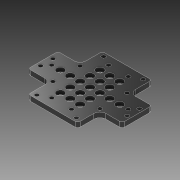
# Autodesk Inventor part: Drill Guide
Saved by Autodesk Inventor 2022 (Build 260153000, 153)
## iProperties
Created: 2021-07-10
Part Number: Drill Guide
Material: Aluminum 6061
Document SubType Name: Modeling
Designer: Max Boord
Density: 2.7 g/cm^3
Appearance: Glossy - Black
Author: Max Boord
Autodesk Inventor part; units mm, degrees
ref_plane "YZ Plane" through (0, 0, 0) normal (1, 0, 0) x (0, 1, 0)
ref_plane "XZ Plane" through (0, 0, 0) normal (0, 1, 0) x (-1, 0, 0)
ref_plane "XY Plane" through (0, 0, 0) normal (0, 0, 1) x (1, 0, 0)
sketch "Sketch1" plane through (0, 0, 0) normal (0, 1, 0) x (-1, 0, 0)
  line L0 (-25.4, -38.1) -> (25.4, -38.1) construction
  line L1 (25.4, -38.1) -> (25.4, -29.8901)
  line L2 (25.4, 38.1) -> (-25.4, 38.1) construction
  line L3 (-25.4, -29.8901) -> (-25.4, -38.1)
  line L4 (-25.4, -38.1) -> (25.4, 38.1) construction
  line L5 (25.4, -38.1) -> (-25.4, 38.1) construction
  circle A0 centre (12.7, -28.575) radius 4.7625
  circle A1 centre (0, -28.575) radius 4.7625
  circle A2 centre (-12.7, -28.575) radius 4.7625
  circle A3 centre (12.7, -15.875) radius 4.7625
  circle A4 centre (0, -15.875) radius 4.7625
  circle A5 centre (-12.7, -15.875) radius 4.7625
  circle A6 centre (12.7, -3.175) radius 4.7625
  circle A7 centre (0, -3.175) radius 4.7625
  circle A8 centre (-12.7, -3.175) radius 4.7625
  circle A9 centre (12.7, 9.525) radius 4.7625
  circle A10 centre (0, 9.525) radius 4.7625
  circle A11 centre (-12.7, 9.525) radius 4.7625
  circle A12 centre (12.7, 22.225) radius 4.7625
  circle A13 centre (0, 22.225) radius 4.7625
  circle A14 centre (-12.7, 22.225) radius 4.7625
  line L6 (47.625, -15.875) -> (47.625, 9.525) construction
  circle A15 centre (25.4, -3.175) radius 4.7625
  circle A16 centre (38.1, -3.175) radius 4.7625
  line L7 (0, -38.1) -> (0, 38.1) construction
  circle A17 centre (-25.4, -3.175) radius 4.7625
  circle A18 centre (-38.1, -3.175) radius 4.7625
  arc A19 (39.4151, -15.875) -> (25.4, -29.8901) centre (39.4151, -29.8901) ccw construction
  line L8 (25.4, 38.1) -> (25.4, 23.5401) construction
  arc A20 (25.4, 23.5401) -> (39.4151, 9.525) centre (39.4151, 23.5401) ccw construction
  line L9 (-60.325, -15.875) -> (-39.4151, -15.875) construction
  line L10 (-60.325, 9.525) -> (-39.4151, 9.525) construction
  arc A21 (-25.4, -29.8901) -> (-39.4151, -15.875) centre (-39.4151, -29.8901) ccw construction
  line L11 (-25.4, 23.5401) -> (-25.4, 38.1) construction
  arc A22 (-39.4151, 9.525) -> (-25.4, 23.5401) centre (-39.4151, 23.5401) ccw construction
  line L12 (53.975, -15.875) -> (28.575, -15.875) construction
  line L13 (25.4, -19.05) -> (25.4, -44.45) construction
  line L14 (-25.4, -44.45) -> (-25.4, -19.05) construction
  line L15 (-28.575, -15.875) -> (-39.4151, -15.875) construction
  line L16 (-25.4, 23.5401) -> (-25.4, 12.7) construction
  line L17 (-39.4151, 9.525) -> (-28.575, 9.525) construction
  line L18 (25.4, 23.5401) -> (25.4, 12.7) construction
  line L19 (28.575, 9.525) -> (53.975, 9.525) construction
  arc A23 (25.4, 12.7) -> (28.575, 9.525) centre (28.575, 12.7) ccw construction
  arc A24 (28.575, -15.875) -> (25.4, -19.05) centre (28.575, -19.05) ccw construction
  arc A25 (-25.4, -19.05) -> (-28.575, -15.875) centre (-28.575, -19.05) ccw construction
  arc A26 (-28.575, 9.525) -> (-25.4, 12.7) centre (-28.575, 12.7) ccw construction
  line L20 (39.4151, -22.225) -> (53.975, -22.225)
  line L21 (53.975, -22.225) -> (53.975, 15.875) construction
  line L22 (53.975, 15.875) -> (39.4151, 15.875)
  arc A27 (39.4151, -22.225) -> (31.75, -29.8901) centre (39.4151, -29.8901) ccw
  line L23 (31.75, -29.8901) -> (31.75, -44.45)
  line L24 (31.75, -44.45) -> (-31.75, -44.45) construction
  line L25 (-31.75, -44.45) -> (-31.75, -29.8901)
  arc A28 (-31.75, -29.8901) -> (-39.4151, -22.225) centre (-39.4151, -29.8901) ccw
  line L26 (-39.4151, -22.225) -> (-60.325, -22.225)
  line L27 (-60.325, -22.225) -> (-60.325, 15.875)
  line L28 (-60.325, 15.875) -> (-39.4151, 15.875)
  arc A29 (-39.4151, 15.875) -> (-31.75, 23.5401) centre (-39.4151, 23.5401) ccw
  line L29 (-31.75, 23.5401) -> (-31.75, 44.45)
  line L30 (-31.75, 44.45) -> (31.75, 44.45)
  line L31 (31.75, 44.45) -> (31.75, 23.5401)
  arc A30 (31.75, 23.5401) -> (39.4151, 15.875) centre (39.4151, 23.5401) ccw
  line L32 (25.4, 38.1) -> (25.4, 44.45) construction
  line L33 (-25.4, 38.1) -> (-25.4, 44.45)
  circle A31 centre (-55.5625, -3.175) radius 4.7625 construction
  circle A32 centre (49.2125, -3.175) radius 4.7625 construction
  circle A33 centre (0, -39.6875) radius 4.7625 construction
  circle A34 centre (0, 39.6875) radius 4.7625 construction
  line L34 (44.45, -17.4132) -> (44.45, -3.2681) construction
  line L35 (-50.8, -20.963) -> (-50.8, -1.2168) construction
  line L36 (-5.6388, -34.925) -> (9.5526, -34.925) construction
  line L37 (-7.9375, 34.925) -> (9.5526, 34.925) construction
  circle A35 centre (-55.5625, -3.175) radius 2.4892 construction
  circle A36 centre (0, -39.6875) radius 2.4892 construction
  circle A37 centre (49.2125, -3.175) radius 2.4892
  circle A38 centre (0, 39.6875) radius 2.4892 construction
  line L38 (33.9951, -24.4701) -> (26.3299, -16.8049) construction
  circle A39 centre (30.1625, -20.6375) radius 2.5527
  circle A40 centre (-30.1625, -20.6375) radius 2.5527
  line L39 (53.975, -3.175) -> (-60.325, -3.175) construction
  circle A41 centre (30.1625, 14.2875) radius 2.5527
  circle A42 centre (-30.1625, 14.2875) radius 2.5527
  circle A43 centre (25.4, 39.6875) radius 2.4892
  circle A44 centre (12.7, 39.6875) radius 2.4892 construction
  circle A45 centre (0, 39.6875) radius 2.4892 construction
  circle A46 centre (-12.7, 39.6875) radius 2.4892 construction
  circle A47 centre (-25.4, 39.6875) radius 2.4892
  circle A48 centre (12.7, -39.6875) radius 2.4892
  circle A49 centre (25.4, -39.6875) radius 2.4892 construction
  circle A50 centre (-12.7, -39.6875) radius 2.4892
  circle A51 centre (-25.4, -39.6875) radius 2.4892 construction
  circle A52 centre (49.2125, -11.1125) radius 2.4892 construction
  circle A53 centre (30.1625, -20.6375) radius 4.7625 construction
  circle A54 centre (49.2125, 4.7625) radius 2.4892 construction
  circle A55 centre (49.2125, 4.7625) radius 4.7625 construction
  circle A56 centre (49.2125, -11.1125) radius 4.7625 construction
  circle A57 centre (-55.5625, -11.1125) radius 2.4892
  circle A58 centre (-55.5625, -11.1125) radius 4.7625 construction
  circle A59 centre (-55.5625, 4.7625) radius 2.4892
  circle A60 centre (-55.5625, 4.7625) radius 4.7625 construction
  circle A61 centre (-12.7, 33.3375) radius 2.4892
  circle A62 centre (12.7, 33.3375) radius 2.4892
  circle A63 centre (-25.4, -46.0375) radius 2.4892
  circle A64 centre (25.4, -46.0375) radius 2.4892
  line L40 (31.75, -44.45) -> (31.75, -50.8)
  line L41 (31.75, -50.8) -> (-31.75, -50.8)
  line L42 (-31.75, -50.8) -> (-31.75, -44.45)
  line L43 (25.4, -44.45) -> (25.4, -50.8) construction
  line L44 (-25.4, -44.45) -> (-25.4, -50.8) construction
  circle A65 centre (-49.2125, -3.175) radius 2.4892
  circle A66 centre (55.5625, 4.7625) radius 2.4892
  circle A67 centre (55.5625, -11.1125) radius 2.4892
  line L45 (53.975, -22.225) -> (60.325, -22.225)
  line L46 (60.325, -22.225) -> (60.325, 15.875)
  line L47 (53.975, 15.875) -> (60.325, 15.875)
  line L48 (53.975, 9.525) -> (60.325, 9.525) construction
  line L49 (53.975, -15.875) -> (60.325, -15.875) construction
  circle A68 centre (25.4, -46.0375) radius 4.7625
  line L50 (25.4, -41.275) -> (19.287, -41.275)
  circle A69 centre (12.7, 33.3375) radius 4.7625
  line L51 (15.952, 28.575) -> (5.0903, 28.575) construction
  circle A70 centre (55.5625, 4.7625) radius 4.7625 construction
  line L52 (50.8, 8.631) -> (50.8, -0.466) construction
  point P0 (0, 0)
  point P1 (47.625, -3.175)
  point P2 (-25.4, 9.525)
  point P3 (47.625, -15.875)
  point P4 (47.625, 9.525)
  dimension "d15" = 25.4
  dimension "d0" = 50.8
  dimension "d3" = 9.525
  dimension "d6" = 12.7
  dimension "d9" = 12.7
  dimension "d18" = 12.7
  dimension "d29" = 3.175
  dimension "d30" = 6.35
  dimension "d31" = 7.6651
  dimension "d65" = 9.525
  dimension "d67" = 6.35
  dimension "d68" = 12.7
  dimension "d69" = 4.7625
  dimension "d70" = 25.4
  dimension "d71" = 6.35
  dimension "d74" = 12.7
  dimension "d89" = 4.9784
  dimension "d90" = 5.1054
  dimension "d100" = 4.9784
  dimension "d101" = 6.35
  dimension "d104" = 12.7
  dimension "d112" = 360
  dimension "d114" = 4.9784
  dimension "d126" = 9.525
  dimension "d127" = 9.525
  dimension "d128" = 9.525
  dimension "d129" = 4.9784
  dimension "d132" = 360
  dimension "d134" = 47.625
  dimension "d135" = 47.625
  dimension "d138" = 360
  dimension "d140" = 60.325
  dimension "d141" = 60.325
  dimension "d142" = 6.35
  dimension "d143" = 12.7
  constraints: 106 end point, 70 centre point, 39 tangent, 27 point on circle, 26 point on line, 20 equal radius, 18 horizontal, 13 coincident, 13 perpendicular, 13 vertical, 8 midpoint, 5 parallel, 5 symmetric about line, 4 horizontal alignment, 2 vertical alignment, 109 other
  measures "d0" distance of L2.end L2.start
  measures "d3" diameter of A0
  measures "d6" distance of A0.centre A1.centre
  measures "d9" distance of A0.centre A3.centre
  measures "d18" distance of A6.centre A15.centre
  measures "d29" radius of A23
  measures "d31" radius of A29
  measures "d65" diameter of A31
  measures "d67" distance from line of A16.centre L34
  measures "d68" distance from line of A18.centre L35
  measures "d69" distance from line of A31.centre L27
  measures "d70" distance between parallel lines of L10 L9
  measures "d71" distance from line of A1.centre L36
  measures "d74" distance from line of A13.centre L37
  measures "d89" diameter of A35
  measures "d90" diameter of A39
  measures "d100" diameter of A43
  measures "d101" distance from line of A43.centre L31
  measures "d104" distance of A43.centre A44.centre
  measures "d114" diameter of A52
  measures "d126" diameter of A53
  measures "d127" diameter of A34
  measures "d128" diameter of A32
  measures "d129" diameter of A57
  measures "d134" distance from line of L30 A7.centre
  measures "d135" distance from line of L41 A7.centre
  measures "d140" distance from line of L27 A7.centre
  measures "d141" distance from line of point (0, 0) L46
  measures "d142" distance from line of L51 A12.centre
  measures "d143" distance from line of L52 A16.centre
extrude "Extrusion1" add sketch "Sketch1" along normal blind 6.35 contours A68 | A27 L23 L40 L41 L42 L25 A28 L26 L27 L28 A29 L29 L30 L31 A30 L22 L47 L46 L45 L20 | A69
sketch "Sketch2" plane through (0, 0, 0) normal (0, -1, 0) x (1, 0, 0)
  circle A0 centre (38.1, -3.175) radius 4.7625 projected
  circle A1 centre (25.4, -3.175) radius 4.7625 projected
  circle A2 centre (12.7, -28.575) radius 4.7625 projected
  circle A3 centre (12.7, -15.875) radius 4.7625 projected
  circle A4 centre (12.7, -3.175) radius 4.7625 projected
  circle A5 centre (12.7, 9.525) radius 4.7625 projected
  circle A6 centre (12.7, 22.225) radius 4.7625 projected
  circle A7 centre (0, 22.225) radius 4.7625 projected
  circle A8 centre (-12.7, 22.225) radius 4.7625 projected
  circle A9 centre (-25.4, -3.175) radius 4.7625 projected
  circle A10 centre (-38.1, -3.175) radius 4.7625 projected
  circle A11 centre (-12.7, 9.525) radius 4.7625 projected
  circle A12 centre (0, 9.525) radius 4.7625 projected
  circle A13 centre (0, -28.575) radius 4.7625 projected
  circle A14 centre (-12.7, -28.575) radius 4.7625 projected
  circle A15 centre (0, -15.875) radius 4.7625 projected
  circle A16 centre (-12.7, -15.875) radius 4.7625 projected
  circle A17 centre (0, -3.175) radius 4.7625 projected
  circle A18 centre (-12.7, -3.175) radius 4.7625 projected
  point P0 (0, 0)
  point P1 (38.1, -3.175)
  point P2 (25.4, -3.175)
  point P3 (12.7, -28.575)
  point P4 (12.7, -15.875)
  point P5 (12.7, -3.175)
  point P6 (12.7, 9.525)
  point P7 (12.7, 22.225)
  point P8 (0, 22.225)
  point P9 (-12.7, 22.225)
  point P10 (-25.4, -3.175)
  point P11 (-38.1, -3.175)
  point P12 (-12.7, 9.525)
  point P13 (0, 9.525)
  point P14 (0, -28.575)
  point P15 (-12.7, -28.575)
  point P16 (0, -15.875)
  point P17 (-12.7, -15.875)
  point P18 (0, -3.175)
  point P19 (-12.7, -3.175)
  constraints: 19 coincident
hole "Hole1" at (38.1, 0, -3.175) at (25.4, 0, -3.175) at (12.7, 0, -28.575) at (12.7, 0, -15.875) at (12.7, 0, -3.175) at (12.7, 0, 9.525) at (12.7, 0, 22.225) at (0, 0, 22.225) at (-12.7, 0, 22.225) at (-25.4, 0, -3.175) at (-38.1, 0, -3.175) at (-12.7, 0, 9.525) at (0, 0, 9.525) at (0, 0, -28.575) at (-12.7, 0, -28.575) at (0, 0, -15.875) at (-12.7, 0, -15.875) at (0, 0, -3.175) at (-12.7, 0, -3.175) direction (0, 1, 0) diameter 9.525 depth 9.525 counterbore diameter 11.9888 counterbore depth 1.524
fillet "Fillet1" radius 3.175 8 edges at (-31.75, 3.175, 44.45) (60.325, 3.175, 15.875) (31.75, 3.175, 44.45) (60.325, 3.175, -22.225) (-31.75, 3.175, -50.8) (31.75, 3.175, -50.8) (-60.325, 3.175, 15.875) (-60.325, 3.175, -22.225)
equation "\"adder\" = d30"
body "Solid1"
